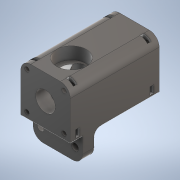
# Autodesk Inventor part: Jorgegrande
Saved by Autodesk Inventor 2020.2 (Build 242310000, 310)
## iProperties
Created: 2021-01-07
Part Number: Jorgegrande
Material: Generic
Document SubType Name: Modeling
Designer: jiali
Density: 1 g/cm^3
Appearance: Default
Author: jiali
Autodesk Inventor part; units mm, degrees
ref_plane "YZ Plane" through (0, 0, 0) normal (1, 0, 0) x (0, 1, 0)
ref_plane "XZ Plane" through (0, 0, 0) normal (0, 1, 0) x (-1, 0, 0)
ref_plane "XY Plane" through (0, 0, 0) normal (0, 0, 1) x (1, 0, 0)
sketch "E" plane through (0, 0, 0) normal (0, 0, 1) x (1, 0, 0)
  line L0 (-20, -20) -> (20, -20)
  line L1 (-20, -20) -> (20, -20)
  line L2 (20, -20) -> (20, 20)
  line L3 (20, 20) -> (-20, 20)
  line L4 (-20, 20) -> (-20, -20)
  circle A0 centre (-15, 15) radius 1.8
  line L5 (-15, 15) -> (-15, 16.8)
  circle A1 centre (15, 15) radius 1.8
  line L6 (15, 15) -> (15, 16.8)
  circle A2 centre (15, -15) radius 1.8
  line L7 (15, -15) -> (15, -13.2)
  circle A3 centre (-15, -15) radius 1.8
  line L8 (-15, -15) -> (-15, -13.2)
  circle A4 centre (0, 0) radius 7.9648
  circle A5 centre (0, 0) radius 8
  circle A6 centre (0, 0) radius 5.1
  dimension "d2" = 40
  constraints: 18 end point, 4 vertical alignment, 3 centre point, 3 coincident, 3 perpendicular, 1 collinear, 1 point on line, 8 other
  measures "d2" distance of L0.end L2.end
extrude "Extrusion1" add sketch "E" against normal blind 72 contours L4 L3 L2 L0
sketch "Sketch2" plane through (0, 0, 0) normal (0, 0, 1) x (1, 0, 0)
  circle A0 centre (0, 0) radius 5.1
  circle A1 centre (0, 0) radius 8
  circle A2 centre (0, 0) radius 8 projected
  dimension "d5" = 10.2
  dimension "d6" = 16
  constraints: 2 centre point, 2 concentric, 1 coincident
  measures "d5" diameter of A0
  measures "d6" diameter of A1
extrude "Extrusion2" add sketch "Sketch2" against normal blind 72
fillet "Fillet1" radius 8 2 edges at (20, 20, -36) (-20, 20, -36)
sketch "Sketch3" plane through (0, 0, 0) normal (0, 0, 1) x (1, 0, 0)
  circle A0 centre (0, 0) radius 8
  circle A1 centre (0, 0) radius 5.1 projected
  dimension "d9" = 16
  constraints: 1 centre point, 1 coincident, 1 concentric
  measures "d9" diameter of A0
extrude "Extrusion3" cut sketch "Sketch3" against normal blind 11
sketch "Sketch4" plane through (0, 0, -72) normal (0, 0, -1) x (-1, 0, 0)
  circle A0 centre (0, 0) radius 13.3
  dimension "d13" = 26.6
  constraints: 1 centre point, 1 coincident
  measures "d13" diameter of A0
extrude "Extrusion4" cut sketch "Sketch4" against normal blind 9
fillet "Fillet2" radius 2 1 edges at (13.3, 0, -72)
sketch "Sketch5" plane through (-20, -20, 0) normal (0, -1, 0) x (1, 0, 0)
  line L0 (40, 0) -> (40, -72) projected
  line L1 (40, 0) -> (0, 0)
  line L2 (0, 0) -> (0, -10)
  line L3 (0, -10) -> (40, -10)
  line L4 (40, -10) -> (40, 0)
  line L5 (40, -10) -> (0, -10)
  line L6 (0, -10) -> (0, -20)
  line L7 (0, -20) -> (40, -20)
  line L8 (40, -20) -> (40, -10)
  point P0 (20, 0)
  point P1 (40, -20)
  dimension "d17" = 40
  dimension "d18" = 10
  dimension "d19" = 40
  dimension "d20" = 10
  constraints: 16 end point, 4 parallel, 2 horizontal, 2 perpendicular
  measures "d17" distance of L3.end L2.end
  measures "d18" distance of L2.end L1.end
  measures "d19" distance of L7.end L6.end
  measures "d20" distance of L6.end L5.end
extrude "Extrusion5" add sketch "Sketch5" along normal blind 20 contours L0 L7 L6 L3
sketch "Sketch6" plane through (-20, -20, -10) normal (0, 0, 1) x (1, 0, 0)
  line L0 (0, -20) -> (40, -20) projected
  line L1 (0, -20) -> (6, -20)
  line L2 (6, -20) -> (6, -10)
  line L3 (6, -10) -> (0, -10)
  line L4 (0, -10) -> (0, -20)
  circle A0 centre (6, -10) radius 2.75
  circle A1 centre (20, -10) radius 2.75
  circle A2 centre (34, -10) radius 2.75
  point P0 (20, 20)
  dimension "d23" = 6
  dimension "d24" = 10
  dimension "d25" = 5.5
  dimension "d31" = 14
  constraints: 8 end point, 3 centre point, 2 horizontal, 2 parallel, 1 coincident, 1 perpendicular, 4 other
  measures "d23" distance of L3.end L2.end
  measures "d24" distance of L2.end L1.end
  measures "d25" diameter of A0
  measures "d31" distance of A0.centre A1.centre
extrude "Extrusion6" cut sketch "Sketch6" against normal blind 20 contours A0 L3 L2 | L2 L3 A0 | A1 | A2
fillet "Fillet3" radius 5 1 edges at (0, -20, -20)
sketch "Sketch7" plane through (-20, -20, -72) normal (0, -1, 0) x (1, 0, 0)
  line L0 (40, 72) -> (40, 0) projected
  line L1 (40, 0) -> (20, 0)
  line L2 (20, 0) -> (20, 18)
  line L3 (20, 18) -> (40, 18)
  line L4 (40, 18) -> (40, 0)
  circle A0 centre (20, 18) radius 6.75
  point P0 (20, 72)
  dimension "d36" = 20
  dimension "d37" = 18
  dimension "d38" = 13.5
  constraints: 8 end point, 2 parallel, 1 centre point, 1 coincident, 1 horizontal, 1 perpendicular
  measures "d36" distance of L2.end L3.end
  measures "d37" distance of L1.end L2.end
  measures "d38" diameter of A0
extrude "Extrusion7" cut sketch "Sketch7" against normal blind 20 contours A0 L2 L3 | L3 L2 A0
sketch "Sketch8" plane through (-12, 20, 0) normal (0, 1, 0) x (1, 0, 0)
  line L0 (12, 0) -> (12, 21)
  line L1 (12, 0) -> (33, 0) construction
  circle A0 centre (12, 21) radius 12
  circle A1 centre (12, 21) radius 7.9765
  line L2 (0, 0) -> (0, 72) projected
  line L3 (24, 0) -> (0, 0) projected
  line L4 (24, 72) -> (24, 0) projected
  line L5 (0, 72) -> (24, 72) projected
  dimension "d41" = 21
  dimension "d42" = 90
  dimension "d43" = 24
  dimension "d46" = 15.953
  constraints: 4 end point, 2 centre point, 2 coincident, 1 horizontal, 1 perpendicular, 1 vertical
  measures "d41" distance of L0.start L0.end
  measures "d42" angle of L1 L0
  measures "d43" diameter of A0
  measures "d46" diameter of A1
extrude "Extrusion21" add sketch "Sketch6" against normal up to surface (10 mm away) contours A1
sketch "Sketch30" plane through (-12, 20, 0) normal (0, 1, 0) x (1, 0, 0)
  line L0 (12, 0) -> (12, 21)
  line L1 (12, 0) -> (33, 0) construction
  circle A0 centre (12, 21) radius 5.25
  dimension "d118" = 21
  dimension "d119" = 90
  dimension "d120" = 10.5
  constraints: 4 end point, 1 centre point, 1 coincident, 1 horizontal, 1 perpendicular, 1 vertical
  measures "d118" distance of L0.start L0.end
  measures "d119" angle of L1 L0
  measures "d120" diameter of A0
extrude "Extrusion22" cut sketch "Sketch30" against normal blind 20
chamfer "Chamfer1" distance 8.5 angle 60 1 edges at (-5.25, 20, -21) measured on face at (-5.75, 20, -21)
extrude "Extrusion12" cut sketch "Sketch8" against normal blind 10 contours A0
sketch "Sketch17" plane through (0, 10, -21) normal (0, 1, 0) x (1, 0, 0)
  circle A0 centre (0, 0) radius 5.25
  circle A1 centre (0, 0) radius 7.9765
  line L0 (-5.1, 5.2487) -> (5.1, 5.2487)
  line L1 (5.1, 5.2487) -> (5.1, -5.2487)
  line L2 (5.1, -5.2487) -> (-5.1, -5.2487)
  line L3 (-5.1, -5.2487) -> (-5.1, 5.2487)
  line L4 (-5.1, 5.2487) -> (5.1, -5.2487) construction
  line L5 (5.1, 5.2487) -> (-5.1, -5.2487) construction
  line L6 (0, 0) -> (0, 5.25)
  line L7 (0, 0) -> (5.25, 0) construction
  circle A2 centre (0, 5.25) radius 5.1
  point P0 (0, -21)
  point P1 (5.1, 5.2487)
  point P2 (-5.1, 5.2487)
  dimension "d70" = 5.25
  dimension "d71" = 90
  dimension "d72" = 10.2
  dimension "d75" = 10.2
  constraints: 16 end point, 3 centre point, 2 coincident, 2 horizontal, 2 midpoint, 2 parallel, 2 perpendicular, 1 vertical
  measures "d70" distance of L6.start L6.end
  measures "d71" angle of L7 L6
  measures "d72" diameter of A2
  measures "d75" distance of L1.end L2.end
extrude "Extrusion14" cut sketch "Sketch17" against normal blind 10 contours L1 A0 L3 A2 | A0 A2 L1 | L1 L2 A0 | A2 L6 A0 | A0 L0 A2 | L0 A2 A1 | L2 L3 A0 | L6 A2 A0 | A0 A2 L0 | A1 A2 | A0 L3 A2
sketch "Sketch19" plane through (-12, 20, -72) normal (0, 1, 0) x (1, 0, 0)
  circle A0 centre (12, -51) radius 12
  circle A1 centre (12, -51) radius 13.75
  circle A2 centre (12, -51) radius 12 projected
  circle A3 centre (12, -51) radius 12
  circle A4 centre (12, -51) radius 12
  point P0 (12, -72)
  constraints: 4 centre point, 3 coincident, 3 concentric
extrude "Extrusion15" add sketch "Sketch19" against normal blind 10
sketch "Sketch21" plane through (0, 0, 0) normal (0, 0, 1) x (1, 0, 0)
  arc A0 (20, 12) -> (12, 20) centre (12, 12) ccw projected
  line L0 (12, 20) -> (-12, 20) projected
  arc A1 (-12, 20) -> (-20, 12) centre (-12, 12) ccw projected
  line L1 (20, 12) -> (25.5044, 34.4365)
  line L2 (25.5044, 34.4365) -> (-24.1214, 34.7179)
  line L3 (-24.1214, 34.7179) -> (-20, 12)
  point P0 (0, 0)
  constraints: 6 end point
extrude "Extrusion16" cut sketch "Sketch21" against normal blind 100
fillet "Fillet4" radius 8 2 edges at (-20, -40, -15) (20, -40, -15)
sketch "Sketch23" plane through (-12, 20, 0) normal (0, 1, 0) x (1, 0, 0)
  line L0 (24, 0) -> (30, 0)
  line L1 (28.8, 0) -> (25.2, 0) projected
  line L2 (30, 0) -> (34.5, 0) construction
  line L3 (30, 4.5) -> (24, 4.5)
  line L4 (24, 4.5) -> (24, 7.5)
  line L5 (24, 7.5) -> (30, 7.5)
  line L6 (30, 7.5) -> (30, 4.5)
  arc A0 (0, 21) -> (24, 21) centre (12, 21) ccw projected
  line L7 (-6, 4.5) -> (0, 4.5)
  line L8 (0, 4.5) -> (0, 7.5)
  line L9 (0, 7.5) -> (-6, 7.5)
  line L10 (-6, 7.5) -> (-6, 4.5)
  line L11 (30, 64.5) -> (24, 64.5)
  line L12 (24, 64.5) -> (24, 67.5)
  line L13 (24, 67.5) -> (30, 67.5)
  line L14 (30, 67.5) -> (30, 64.5)
  line L15 (-6, 64.5) -> (0, 64.5)
  line L16 (0, 64.5) -> (0, 67.5)
  line L17 (0, 67.5) -> (-6, 67.5)
  line L18 (-6, 67.5) -> (-6, 64.5)
  point P0 (12, 0)
  point P1 (3.9215, 32.1266)
  point P2 (20.0785, 32.1266)
  dimension "d83" = 4.5
  dimension "d85" = 3
  dimension "d88" = 60
  constraints: 36 end point, 2 collinear, 1 horizontal, 1 vertical, 15 other
  measures "d83" distance of L0.end L3.start
  measures "d85" distance of L3.end L4.end
  measures "d88" distance of L3.start L11.start
extrude "Extrusión Tuercas" cut sketch "Sketch23" against normal blind 8.5
sketch "Sketch29" plane through (-20, -20, 0) normal (-1, 0, 0) x (0, 0, 1)
  line L0 (0, 0) -> (-10, 0) projected
  line L1 (0, 0) -> (-6, 0)
  line L2 (-6, 0) -> (-6, 5)
  line L3 (-6, 5) -> (0, 5)
  line L4 (0, 5) -> (0, 0)
  line L5 (-4.5, 8) -> (-7.5, 8)
  line L6 (-7.5, 8) -> (-7.5, 2)
  line L7 (-7.5, 2) -> (-4.5, 2)
  line L8 (-4.5, 2) -> (-4.5, 8)
  line L9 (-4.5, 8) -> (-7.5, 2) construction
  line L10 (-7.5, 8) -> (-4.5, 2) construction
  point P0 (0, 20)
  dimension "d101" = 6
  dimension "d102" = 5
  dimension "d103" = 3
  dimension "d104" = 6
  constraints: 20 end point, 4 parallel, 2 horizontal, 2 midpoint, 2 perpendicular
  measures "d101" distance of L2.end L3.end
  measures "d102" distance of L1.end L2.end
  measures "d103" distance of L7.end L6.end
  measures "d104" distance of L6.end L5.end
extrude "Extrusion20" cut sketch "Sketch29" against normal blind 9 contours L7 L6 L5 L8 L3 L2 | L2 L3 L8 L7
mirror "Mirror1" about plane through (0, 0, 0) normal (1, 0, 0) of "Extrusion20"
ref_plane "Work Plane2" through (0, 0, -36) normal (0, 0, -1) x (-1, 0, 0)
mirror "Mirror2" about plane through (0, 0, -36) normal (0, 0, -1) of "Extrusión Tuercas", "Extrusion20", "Mirror1"
fillet "Fillet5" radius 1 12 edges at (20, -21.4645, -21.4645) (20, -28.5, -20) (17.6569, -37.6569, -20) (0, -40, -20) (-17.6569, -37.6569, -20) (-20, -28.5, -20) (-20, -21.4645, -21.4645) (-20, -20, -48.5) (20, -20, -48.5) (-20, -20, -5) (0, -20, 0) (20, -20, -5)
ref_plane "Work Plane1" through (0, 0, 0) normal (1, 0, 0) x (0, 1, 0)
ref_plane "Work Plane3" through (0, 0, -72) normal (-1, 0, 0) x (0, 1, 0)
ref_plane "Work Plane4" through (0, 0, -72) normal (-1, 0, 0) x (0, 1, 0)
body "Solid1"
